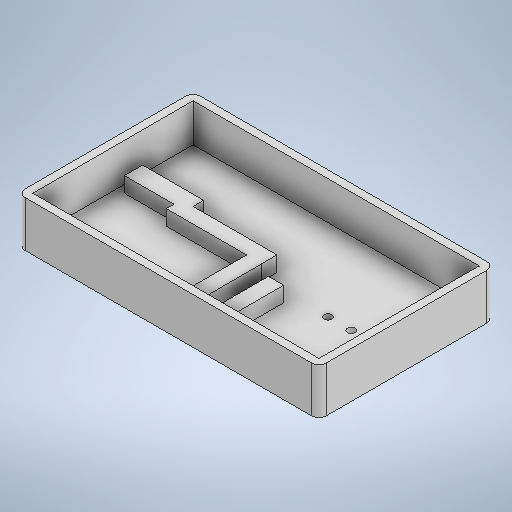
# Autodesk Inventor part: SimpleElectronicBox
Saved by Autodesk Inventor 2025.2 (Build 292293000, 293)
## iProperties
Created: 2026-02-18
Part Number: SimpleElectronicBox
Material: Generic
Document SubType Name: Modeling
Designer: sanku
Density: 1 g/cm^3
Appearance: Default
Author: sanku
Autodesk Inventor part; units mm, degrees
ref_plane "YZ Plane" through (0, 0, 0) normal (1, 0, 0) x (0, 1, 0)
ref_plane "XZ Plane" through (0, 0, 0) normal (0, 1, 0) x (-1, 0, 0)
ref_plane "XY Plane" through (0, 0, 0) normal (0, 0, 1) x (1, 0, 0)
sketch "Sketch1" plane through (0, 0, 0) normal (0, 1, 0) x (-1, 0, 0)
  line L0 (0, 0) -> (-238.125, 0)
  line L1 (-238.125, 0) -> (-238.125, -133.35)
  line L2 (-238.125, -133.35) -> (0, -133.35)
  line L3 (0, -133.35) -> (0, 0)
  line L4 (0, 6.35) -> (-237.998, 6.35)
  line L5 (-244.475, -0.127) -> (-244.475, -133.35)
  line L6 (-238.125, -139.7) -> (-0.1245, -139.7)
  line L7 (6.35, -133.35) -> (6.35, 0)
  arc A0 (-0.1245, -139.7) -> (6.35, -133.35) centre (-0.1245, -133.2243) ccw
  arc A1 (6.35, 0) -> (-0.1245, 6.35) centre (-0.1258, -0.127) ccw
  arc A2 (-244.475, -133.2243) -> (-238.125, -139.7) centre (-237.998, -133.2242) ccw
  arc A3 (-237.998, 6.35) -> (-244.475, -0.127) centre (-237.998, -0.127) ccw
  dimension "d0" = 238.125
  dimension "d1" = 133.35
  dimension "d2" = 6.35
  dimension "d9" = 6.477
  dimension "d10" = 6.477
  dimension "d11" = 6.477
  constraints: 16 end point, 8 point on circle, 5 point on line, 4 centre point, 4 parallel, 2 perpendicular, 1 horizontal, 1 tangent
  measures "d0" distance of L2.end L1.end
  measures "d1" distance of L1.end L0.end
  measures "d2" distance between parallel lines of L3 L7
  measures "d9" radius of A1
  measures "d10" radius of A2
  measures "d11" radius of A3
extrude "Extrusion1" add sketch "Sketch1" along normal blind 38.1
sketch "Sketch2" plane through (0, 0, 0) normal (0, -1, 0) x (1, 0, 0)
  line L0 (0, 0) -> (238.125, 0)
  line L1 (238.125, 0) -> (238.125, -133.35)
  line L2 (238.125, -133.35) -> (0, -133.35)
  line L3 (0, -133.35) -> (0, 0)
  dimension "d5" = 238.125
  dimension "d6" = 133.35
  constraints: 8 end point, 2 parallel, 1 horizontal, 1 perpendicular
  measures "d5" distance of L1.end L2.end
  measures "d6" distance of L0.end L1.end
extrude "Extrusion2" add sketch "Sketch2" against normal blind 6.35
sketch "Sketch7" plane through (0, 6.35, 0) normal (0, 1, 0) x (1, 0, 0)
  line L0 (237.998, 0) -> (155.448, 0)
  line L1 (238.125, 0) -> (0, 0) projected
  line L2 (155.448, 0) -> (155.448, 57.15)
  line L3 (155.448, 57.15) -> (237.998, 57.15)
  circle A0 centre (218.3382, 65.3946) radius 3.175
  circle A1 centre (199.6313, 65.4249) radius 3.175
  line L4 (218.3382, 65.3946) -> (180.2382, 65.3946)
  circle A2 centre (180.2382, 65.3946) radius 3.175
  dimension "d31" = 82.55
  dimension "d32" = 57.15
  dimension "d33" = 6.35
  dimension "d36" = 6.35
  dimension "d37" = 38.1
  dimension "d38" = 6.35
  constraints: 8 end point, 3 centre point, 2 perpendicular, 1 horizontal, 1 point on line
  measures "d31" distance of L0.start L0.end
  measures "d32" distance of L0.end L2.end
  measures "d33" diameter of A0
  measures "d36" diameter of A1
  measures "d37" distance of L4.start L4.end
  measures "d38" diameter of A2
extrude "Extrusion4" cut sketch "Sketch7" against normal blind 6.35
sketch "Sketch11" plane through (0, 6.35, 0) normal (0, 1, 0) x (1, 0, 0)
  line L0 (57.15, 78.6953) -> (0, 78.6953)
  line L1 (47.625, 76.2) -> (127, 76.2) projected
  line L2 (47.625, 76.2) -> (127, 76.2)
  line L3 (127, 76.2) -> (127, 63.5)
  line L4 (127, 63.5) -> (47.625, 63.5)
  line L5 (47.625, 63.5) -> (47.625, 76.2)
  line L6 (114.4338, 63.5) -> (127.1338, 63.5)
  line L7 (127.1338, 63.5) -> (127.1338, 0)
  line L8 (127.1338, 0) -> (114.4338, 0)
  line L9 (114.4338, 0) -> (114.4338, 63.5)
  line L10 (238.125, 0) -> (0, 0) projected
  line L11 (0, 0) -> (0, 82.55)
  line L12 (0, 0) -> (0, 133.35) projected
  line L13 (0, 82.55) -> (57.15, 82.55)
  line L14 (57.15, 82.55) -> (57.15, 0)
  line L15 (0, 78.6953) -> (47.625, 78.6953)
  line L16 (47.625, 78.6953) -> (47.625, 69.85)
  line L17 (47.625, 69.85) -> (0, 69.85)
  line L18 (0, 69.85) -> (0, 78.6953)
  line L19 (57.15, 78.6953) -> (0, 78.6953)
  line L20 (0, 78.6953) -> (0, 85.0453)
  line L21 (0, 85.0453) -> (57.15, 85.0453)
  line L22 (57.15, 85.0453) -> (57.15, 78.6953)
  point P0 (0, 97.7453)
  point P1 (0, 69.85)
  dimension "d59" = 79.375
  dimension "d60" = 12.7
  dimension "d61" = 12.7
  dimension "d62" = 63.5
  dimension "d70" = 82.55
  dimension "d71" = 6.35
  constraints: 40 end point, 8 parallel, 5 horizontal, 5 perpendicular, 3 point on line, 1 midpoint
  measures "d59" distance of L3.end L4.end
  measures "d60" distance of L2.end L3.end
  measures "d61" distance of L7.end L8.end
  measures "d62" distance of L6.end L7.end
  measures "d70" distance of L10.end L11.end
  measures "d71" distance of L19.end L20.end
extrude "Extrusion7" add sketch "Sketch11" along normal blind 12.7 contours L0 L11 L13 L14 | L16 L5 L17 L11 L0 | L13 L12 L21 L22 | L14 L4 L5 L1 | L1 L3 L4 L14 | L6 L7 L8 L9 L4
sketch "Sketch12" plane through (0, 6.35, 0) normal (0, 1, 0) x (1, 0, 0)
  line L0 (238.125, 0) -> (0, 0) projected
  line L1 (238.125, 0) -> (155.575, 0)
  line L2 (151.6176, 0) -> (151.6176, 57.15)
  line L3 (155.575, 57.15) -> (238.125, 57.15)
  line L4 (238.125, 57.15) -> (238.125, 0)
  line L5 (151.6176, 0) -> (138.9176, 0)
  line L6 (138.9176, 0) -> (138.9176, 57.15)
  line L7 (138.9176, 57.15) -> (151.6176, 57.15)
  line L8 (155.575, 57.15) -> (155.575, 0)
  point P0 (151.6176, 57.15)
  point P1 (151.6176, 0)
  dimension "d65" = 82.55
  dimension "d66" = 57.15
  dimension "d67" = 12.7
  constraints: 16 end point, 4 parallel, 2 horizontal, 2 perpendicular
  measures "d65" distance of L3.start L3.end
  measures "d66" distance of L2.start L2.end
  measures "d67" distance of L6.end L7.end
extrude "Extrusion8" add sketch "Sketch12" along normal blind 12.7 contours L0 L6 L7 L2
sketch "Sketch13" plane through (0, 19.05, 0) normal (0, 1, 0) x (1, 0, 0)
  line L0 (0, 85.0453) -> (57.15, 85.0453) projected
  line L1 (47.625, 69.85) -> (0, 69.85) projected
  line L2 (0, 85.0453) -> (6.35, 85.0453)
  line L3 (6.35, 85.0453) -> (6.35, 69.85)
  line L4 (6.35, 69.85) -> (0, 69.85)
  line L5 (0, 69.85) -> (0, 85.0453)
  point P0 (0, 0)
  dimension "d72" = 6.35
  constraints: 8 end point, 2 parallel, 1 horizontal, 1 perpendicular, 1 point on line
  measures "d72" distance of L3.end L4.end
extrude "Extrusion9" cut sketch "Sketch13" against normal blind 12.7
sketch "Sketch14" plane through (0, 19.05, 0) normal (0, 1, 0) x (1, 0, 0)
  line L0 (47.625, 78.6953) -> (47.625, 76.2) projected
  line L1 (47.625, 78.6953) -> (57.15, 78.6953)
  line L2 (57.15, 78.6953) -> (57.15, 76.0675)
  line L3 (57.15, 76.0675) -> (47.625, 76.0675)
  line L4 (47.625, 76.0675) -> (47.625, 78.6953)
  point P0 (0, 0)
  constraints: 8 end point, 2 parallel, 1 horizontal, 1 perpendicular
extrude "Extrusion10" add sketch "Sketch14" against normal blind 12.7
sketch "Sketch15" plane through (0, 19.05, 0) normal (0, 1, 0) x (1, 0, 0)
  point P0 (0, 0)
equation "\"d34\" = d38"
body "Solid1"
